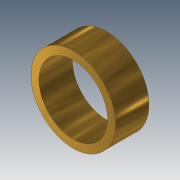
# Autodesk Inventor part: Xfordring
Saved by Autodesk Inventor 2019 (Build 230136000, 136)
## iProperties
Created: 2019-01-12
Part Number: Xfordring
Material: Brass, Soft Yellow
Document SubType Name: Modeling
Designer: LillaHunden
Density: 8.47 g/cm^3
Appearance: Brass - Satin
Author: LillaHunden
Autodesk Inventor part; units mm, degrees
ref_plane "YZ Plane" through (0, 0, 0) normal (1, 0, 0) x (0, 1, 0)
ref_plane "XZ Plane" through (0, 0, 0) normal (0, 1, 0) x (-1, 0, 0)
ref_plane "XY Plane" through (0, 0, 0) normal (0, 0, 1) x (1, 0, 0)
sketch "Sketch1" plane through (0, 0, 0) normal (0, 0, 1) x (1, 0, 0)
  circle A0 centre (0, 0) radius 3.25
  circle A1 centre (0, 0) radius 4
  dimension "d0" = 6.5
  dimension "d1" = 8
  constraints: 2 centre point, 2 coincident
  measures "d0" diameter of A0
  measures "d1" diameter of A1
ref_plane "Work Plane1" through (-8.6525, -8.6525, -3.172) normal (0, 0, 1) x (0.844775, 0.5351216, 0)
extrude "Extrusion1" add sketch "Sketch1" against normal up to surface (3.172 mm away)
body "Solid1"
